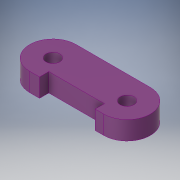
# Autodesk Inventor part: КВ33.044.207 - Прижим ремня
Saved by Autodesk Inventor 2019 (Build 230136000, 136)
## iProperties
Created: 2019-08-18
Part Number: КВ33.044.207 - Прижим ремня
Material: Пластик АБС
Document SubType Name: Modeling
Designer: Петров Иван
Density: 1.06 g/cm^3
Appearance: Гладкий — пурпурный
Author: Петров Иван
Autodesk Inventor part; units mm, degrees
ref_plane "YZ Plane" through (0, 0, 0) normal (1, 0, 0) x (0, 1, 0)
ref_plane "XZ Plane" through (0, 0, 0) normal (0, 1, 0) x (-1, 0, 0)
ref_plane "XY Plane" through (0, 0, 0) normal (0, 0, 1) x (1, 0, 0)
sketch "Эскиз1" plane through (0, 0, 0) normal (0, 1, 0) x (-1, 0, 0)
  circle A0 centre (0, 2.5) radius 0.75
  line L0 (0.9421, 0) -> (0.9421, 5)
  line L1 (0.9421, 5) -> (0, 5)
  arc A1 (0, 5) -> (0, 0) centre (0, 2.5) ccw
  line L2 (0.9421, 0) -> (0, 0)
  line L3 (0.9421, 0) -> (0.9421, 5)
  line L4 (6.9421, 0) -> (0.9421, 0)
  line L5 (6.9421, 5) -> (6.9421, 0)
  line L6 (0.9421, 5) -> (6.9421, 5)
  circle A2 centre (8, 2.5) radius 0.75
  line L7 (6.9421, 5) -> (6.9421, 0)
  line L8 (8, 0) -> (6.9421, 0)
  arc A3 (8, 0) -> (8, 5) centre (8, 2.5) ccw
  line L9 (8, 5) -> (6.9421, 5)
  line L10 (0.9421, 5) -> (6.9421, 5)
  line L11 (6.9421, 5) -> (6.9421, 4)
  line L12 (6.9421, 4) -> (0.9421, 4)
  line L13 (0.9421, 4) -> (0.9421, 5)
  point P0 (4, 5)
  dimension "d0" = 1
  constraints: 28 end point, 4 centre point, 4 point on circle, 2 parallel, 1 horizontal, 1 perpendicular, 1 point on line
  measures "d0" distance of L10.end L11.end
extrude "Выдавливание1" add sketch "Эскиз1" along normal blind 2 contours L2 A1 L1 L0 | L0 L12 L5 L4 | L5 L9 A3 L8
